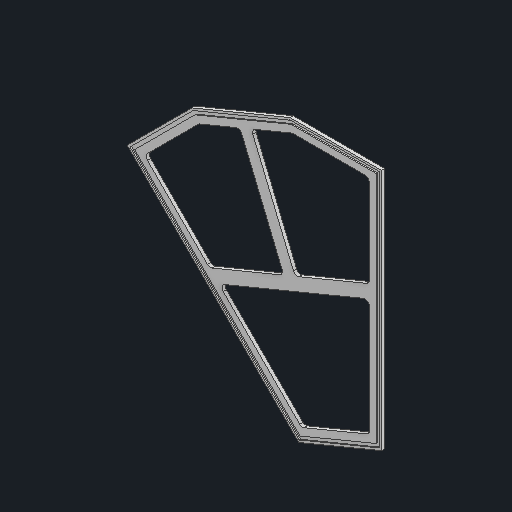
# Autodesk Inventor part: DMF 01 51 outside frame v2.1
Saved by Autodesk Inventor 2026.2 (Build 302298010, 298A)
## iProperties
Created: 2024-05-05
Part Number: DMF 01 51 outside frame v2.1
Material: Generic
Document SubType Name: Modeling
Designer: pokla
Density: 1 g/cm^3
Appearance: Default
Author: pokla
Autodesk Inventor part; units mm, degrees
ref_plane "YZ Plane" through (0, 0, 0) normal (1, 0, 0) x (0, 1, 0)
ref_plane "XZ Plane" through (0, 0, 0) normal (0, 1, 0) x (-1, 0, 0)
ref_plane "XY Plane" through (0, 0, 0) normal (0, 0, 1) x (1, 0, 0)
sketch "Sketch1" plane through (0, 0, 0) normal (0, 0, 1) x (1, 0, 0)
  line L0 (0, 286.8339) -> (202.8222, 202.8222) construction
  line L1 (202.8222, 202.8222) -> (286.8339, 0) construction
  line L2 (286.8339, 0) -> (202.8222, -202.8222) construction
  line L3 (202.8222, -202.8222) -> (0, -286.8339) construction
  line L4 (0, -286.8339) -> (-202.8222, -202.8222) construction
  line L5 (-202.8222, -202.8222) -> (-286.8339, 0) construction
  line L6 (-286.8339, 0) -> (-202.8222, 202.8222) construction
  line L7 (-202.8222, 202.8222) -> (0, 286.8339)
  line L8 (-202.8222, 202.8222) -> (0, 286.8339)
  line L9 (-464.5194, 781.7427) -> (-224.3107, 881.2404)
  line L10 (-101.4111, 244.8281) -> (-344.4151, 831.4916) construction
  line L11 (-224.3107, 881.2404) -> (0, 881.2404)
  line L12 (0, 881.2404) -> (0, 286.8339)
  line L13 (-464.5194, 781.7427) -> (-623.1311, 623.1311)
  line L14 (-623.1311, 623.1311) -> (-202.8222, 202.8222)
  point P0 (0, 0)
  point P1 (0, 0)
  dimension "d0" = 530
  dimension "d2" = 260
  dimension "d3" = 635
  constraints: 30 end point, 2 midpoint, 1 coincident, 1 horizontal, 1 parallel, 1 perpendicular, 1 symmetric about line, 1 vertical, 1 vertical alignment, 17 other
  measures "d0" distance between parallel lines of L5 L1
  measures "d2" distance of L9.start L9.end
  measures "d3" distance of L10.end L10.start
extrude "Extrusion1" add sketch "Sketch1" along normal mid plane 8
sketch "Sketch2" plane through (0, 0, 4) normal (0, 0, 1) x (1, 0, 0)
  line L0 (-224.3107, 881.2404) -> (-464.5194, 781.7427) projected
  line L1 (-464.5194, 781.7427) -> (-623.1311, 623.1311) projected
  line L2 (-239.6414, 539.3487) -> (-421.5665, 463.9929)
  line L3 (-202.8222, 202.8222) -> (0, 286.8339) projected
  line L4 (-101.4111, 244.8281) -> (-344.4151, 831.4916) construction
  line L5 (-623.1311, 623.1311) -> (-202.8222, 202.8222) projected
  line L6 (-421.5665, 463.9929) -> (-580.7047, 623.1311)
  line L7 (-580.7047, 623.1311) -> (-447.5258, 756.31)
  line L8 (-447.5258, 756.31) -> (-346.7928, 798.0349)
  line L9 (-239.6414, 539.3487) -> (-346.7928, 798.0349)
  line L10 (-211.925, 550.8292) -> (-30, 626.185)
  line L11 (-30, 626.185) -> (-30, 851.2404)
  line L12 (-30, 851.2404) -> (-218.3434, 851.2404)
  line L13 (-218.3434, 851.2404) -> (-319.0764, 809.5154)
  line L14 (-211.925, 550.8292) -> (-319.0764, 809.5154)
  line L15 (0, 286.8339) -> (0, 881.2404) projected
  line L16 (-421.5665, 463.9929) -> (-30, 626.185) construction
  line L17 (-398.6054, 441.0319) -> (-30, 593.7132)
  line L18 (-195.7832, 238.2096) -> (-30, 306.8793)
  line L19 (-30, 306.8793) -> (-30, 593.7132)
  line L20 (-195.7832, 238.2096) -> (-398.6054, 441.0319)
  point P0 (0, 0)
  dimension "d11" = 30
  dimension "d12" = 280
  dimension "d13" = 30
  dimension "d14" = 30
  dimension "d15" = 15
  dimension "d21" = 30
  dimension "d22" = 30
  dimension "d23" = 30
  dimension "d24" = 30
  constraints: 32 end point, 5 parallel, 5 symmetric about line, 2 midpoint, 1 collinear
  measures "d11" distance between parallel lines of L5 L6
  measures "d12" distance between parallel lines of L8 L2
  measures "d13" distance between parallel lines of L0 L8
  measures "d14" distance between parallel lines of L1 L7
  measures "d15" distance between parallel lines of L9 L4
  measures "d21" distance between parallel lines of L16 L17
  measures "d22" distance between parallel lines of L5 L20
  measures "d23" distance between parallel lines of L19 L15
  measures "d24" distance between parallel lines of L18 L3
extrude "Extrusion2" cut sketch "Sketch2" against normal up to surface (8 mm away)
fillet "Fillet1" radius 10 12 edges at (-580.7047, 623.1311, 0) (-346.7928, 798.0349, 0) (-239.6414, 539.3487, 0) (-421.5665, 463.9929, 0) (-319.0764, 809.5154, 0) (-30, 851.2404, 0) (-30, 626.185, 0) (-211.925, 550.8292, 0) (-398.6054, 441.0319, 0) (-30, 593.7132, 0) (-30, 306.8793, 0) (-195.7832, 238.2096, 0)
sketch "Sketch4" plane through (0, 0, 4) normal (0, 0, 1) x (1, 0, 0)
  line L0 (-224.3107, 881.2404) -> (-464.5194, 781.7427) projected
  line L1 (0, 881.2404) -> (-224.3107, 881.2404) projected
  line L2 (-464.5194, 781.7427) -> (-623.1311, 623.1311) projected
  line L3 (-623.1311, 623.1311) -> (-202.8222, 202.8222) projected
  line L4 (-202.8222, 202.8222) -> (0, 286.8339) projected
  line L5 (0, 286.8339) -> (0, 881.2404) projected
  line L6 (-461.6872, 777.5039) -> (-223.3162, 876.2404)
  line L7 (-223.3162, 876.2404) -> (-5, 876.2404)
  line L8 (-5, 876.2404) -> (-5, 290.1748)
  line L9 (-5, 290.1748) -> (-201.6491, 208.7201)
  line L10 (-201.6491, 208.7201) -> (-616.06, 623.1311)
  line L11 (-616.06, 623.1311) -> (-461.6872, 777.5039)
  line L12 (-221.7249, 868.2404) -> (-457.1555, 770.7219)
  line L13 (-457.1555, 770.7219) -> (-604.7463, 623.1311)
  line L14 (-604.7463, 623.1311) -> (-199.772, 218.1568)
  line L15 (-199.772, 218.1568) -> (-13, 295.5203)
  line L16 (-13, 295.5203) -> (-13, 868.2404)
  line L17 (-13, 868.2404) -> (-221.7249, 868.2404)
  point P0 (0, 0)
  dimension "d26" = 5
  dimension "d27" = 8
  constraints: 24 end point, 10 other
  measures "d26" distance between parallel lines of L0 L6
  measures "d27" distance between parallel lines of L6 L12
extrude "Extrusion3" cut sketch "Sketch4" against normal blind 3 contours L6 L7 L8 L9 L10 L11
fillet "Fillet3" radius 16 2 edges at (-223.3162, 876.2404, 2.5) (-461.6872, 777.5039, 2.5)
fillet "Fillet4" radius 8 2 edges at (-457.1555, 770.7219, 2.5) (-221.7249, 868.2404, 2.5)
equation "\"d0\" = Барабан_размер_по_плоскостям"
equation "\"d2\" = Кассета_длина_грани"
equation "\"d3\" = Кассета_высота"
equation "\"d11\" = d13"
equation "\"d14\" = d13"
equation "\"d15\" = 0.5 * d13"
equation "\"d21\" = d13"
equation "\"d22\" = d13"
equation "\"d23\" = d13"
equation "\"d24\" = d13"
equation "\"Барабан_размер_по_плоскостям\" = 530"
equation "\"Кассета_длина_грани\" = 260"
equation "\"Кассета_высота\" = 635"
body "Solid1"
